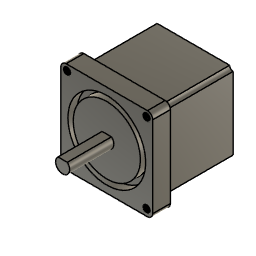
Motor (Autodesk Fusion 360 design; units mm, degrees)
Autodesk Fusion 360 part; units mm, degrees
sketch "Sketch1" plane through (0, 0, 0) normal (0, 1, 0) x (1, 0, 0)
  line L0 (26, 26) -> (-26, 26)
  line L1 (-26, 26) -> (-26, -26)
  line L2 (-26, -26) -> (26, -26)
  line L3 (26, -26) -> (26, 26)
  line L4 (26, 26) -> (-26, -26) construction
  line L5 (-26, 26) -> (26, -26) construction
  circle A0 centre (0, 0) radius 22
  circle A1 centre (0, 0) radius 19
  line L6 (22.5, 22.5) -> (-22.5, 22.5)
  line L7 (-22.5, 22.5) -> (-22.5, -22.5)
  line L8 (-22.5, -22.5) -> (22.5, -22.5)
  line L9 (22.5, -22.5) -> (22.5, 22.5)
  line L10 (22.5, 22.5) -> (-22.5, -22.5) construction
  line L11 (-22.5, 22.5) -> (22.5, -22.5) construction
  circle A2 centre (0, 0) radius 4
  line L12 (-2.6458, -3) -> (2.6458, -3)
  circle A3 centre (-22.5, -22.5) radius 2
  circle A4 centre (22.5, -22.5) radius 2
  circle A5 centre (-22.5, 22.5) radius 2
  circle A6 centre (22.5, 22.5) radius 2
  dimension "d1" = 52
  dimension "d2" = 52
  dimension "d3" = 44
  dimension "d4" = 38
  dimension "d5" = 45
  dimension "d6" = 45
  dimension "d7" = 8
  dimension "d8" = 3
  dimension "d9" = 4
  dimension "d10" = 4
  dimension "d11" = 4
  dimension "d12" = 4
  constraint horizontal L0
  constraint perpendicular L0 L1
  constraint parallel L0 L2
  constraint parallel L1 L3
  constraint coincident L4 A0.centre
  constraint coincident L5 A0.centre
  constraint coincident A0.centre A1.centre
  constraint concentric A0 A1
  constraint horizontal L6
  constraint perpendicular L6 L7
  constraint parallel L6 L8
  constraint parallel L7 L9
  constraint coincident L10 A0.centre
  constraint coincident L11 A0.centre
  constraint concentric A1 A2
  constraint coincident A2 L12.start
  constraint coincident A2 L12.end
  constraint horizontal L12
  constraint coincident L7.end L8.start
  constraint coincident L8.end L9.start
  constraint coincident L6.end L7.start
  constraint coincident L6.start L9.end
  measures "d1" distance of L1.end L2.end
  measures "d2" distance of L0.end L1.end
  measures "d3" diameter of A0
  measures "d4" diameter of A1
  measures "d5" distance of L7.end L8.end
  measures "d6" distance of L6.end L7.end
  measures "d7" diameter of A2
  measures "d8" distance of A0.centre L12
  measures "d9" diameter of A3
  measures "d10" diameter of A4
  measures "d11" diameter of A5
  measures "d12" diameter of A6
extrude "Extrude1" add sketch "Sketch1" along normal blind 44 contours A0 | A1 | L6 L7 L8 L9 A3 A4 A5 A6 | A2 L12 | A2 L12
extrude "Extrude2" add sketch "Sketch1" along normal blind 5 contours L0 L1 L2 L3 | L6 L7 A5 | L6 L7 A5 | L6 L9 A6 | L6 L9 A6 | L7 L8 A3 | L7 L8 A3 | L8 L9 A4 | L8 L9 A4
extrude "Extrude3" add sketch "Sketch1" against normal blind 5 contours L0 L1 L2 L3 | A1 | L6 L7 L8 L9 A3 A4 A5 A6 | A2 L12 | A2 L12
extrude "Extrude4" add sketch "Sketch1" against normal blind 30 contours A2 L12 picked at (0.8135, -0.7197)
thread "Thread1" "ISO Metric profile 4.0 M4x0.7 M4x0.7 6H" major diameter 4.1095 minor diameter 3.332 pitch 0.7 angle 60 modelled right hand crest width 0.193 on face at (-20.5099, -1.6667, 22.6991) crest through (-20.834, -0.175, 22.5)
thread "Thread2" "ISO Metric profile 4.0 M4x0.7 M4x0.7 6H" major diameter 4.1095 minor diameter 3.332 pitch 0.7 angle 60 modelled right hand crest width 0.193 on face at (24.4901, -3.3333, 22.3009) crest through (24.166, -0.175, 22.5)
thread "Thread3" "ISO Metric profile 4.0 M4x0.7 M4x0.7 6H" major diameter 4.1095 minor diameter 3.332 pitch 0.7 angle 60 modelled right hand crest width 0.193 on face at (24.4901, -1.6667, -22.3009) crest through (24.166, -0.175, -22.5)
thread "Thread4" "ISO Metric profile 4.0 M4x0.7 M4x0.7 6H" major diameter 4.1095 minor diameter 3.332 pitch 0.7 angle 60 modelled right hand crest width 0.193 on face at (-20.5099, -1.6667, -22.3009) crest through (-20.834, -0.175, -22.5)
fillet "Fillet1" radius 3 4 edges at (26, 0, 26) (-26, 0, 26) (-26, 0, -26) (26, 0, -26)
